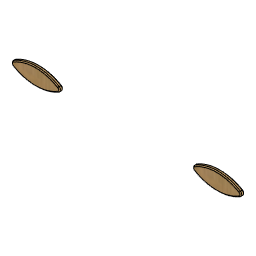
Lamello Bisquit Size 10 Edge SIDE (Autodesk Fusion 360 design; units mm, degrees)
description: Lamello Bisquit
part number: S10
Autodesk Fusion 360 part; units mm, degrees
sketch "Contact Area" plane through (0, 0, 0) normal (0, 0, 1) x (1, 0, 0)
  line L0 (-160, -12.5) -> (160, -12.5)
  line L1 (160, -12.5) -> (160, 12.5)
  line L2 (160, 12.5) -> (-160, 12.5)
  line L3 (-160, 12.5) -> (-160, -12.5)
  line L4 (-160, -12.5) -> (160, 12.5) construction
  line L5 (160, -12.5) -> (-160, 12.5) construction
  dimension "d3" = 320
  dimension "d4" = 25
  constraint horizontal L0
  constraint perpendicular L0 L1
  constraint parallel L0 L2
  constraint parallel L1 L3
  constraint coincident L4 origin
  constraint coincident L5 origin
  measures "d3" distance of L1.end L2.end
  measures "d4" distance of L0.end L1.end
sketch "Egde/SIDE calc" plane through (0, 0, 0) normal (1, 0, 0) x (0, 1, 0)
  line L0 (-50, 18) -> (50, 18)
  line L1 (50, 18) -> (50, 0)
  line L2 (50, 0) -> (-50, 0)
  line L3 (-50, 0) -> (-50, 18)
  line L4 (-50, 18) -> (50, 0) construction
  line L5 (50, 18) -> (-50, 0) construction
  line L6 (12.5, 0) -> (12.5, -40)
  line L7 (12.5, -40) -> (-12.5, -40)
  line L8 (-12.5, -40) -> (-12.5, 0)
  line L9 (-12.5, 0) -> (12.5, 0)
  line L10 (-226.25, 106.25) -> (-213.75, 106.25) construction
  line L11 (-264.0981, 93.7573) -> (-251.5981, 93.7573) construction
  line L12 (-5, 14) -> (5, 14)
  line L13 (5, 14) -> (5, -14)
  line L14 (5, -14) -> (-5, -14)
  line L15 (-5, -14) -> (-5, 14)
  line L16 (-5, 14) -> (5, -14) construction
  line L17 (5, 14) -> (-5, -14) construction
  line L18 (0, -14) -> (0, 14) construction
  line L19 (0, 1.75) -> (0, 22.5) construction
  line L20 (-5, -14) -> (-12.5, -14) construction
  line L21 (0, 0) -> (5, 0) construction
  line L22 (12.5, 0) -> (5, 0) construction
  line L23 (12.5, 0) -> (5, 0) construction
  point P0 (0, 9)
  point P1 (12.5, 0)
  dimension "d20" = 100
  dimension "d21" = 18
  dimension "d23" = 40
  dimension "d24" = 90
  dimension "ReferenceCoord_Calculated" = 12.5
  dimension "OtherSideRefYCoord_Calculated" = 12.5
  dimension "d37" = 12.5
  dimension "d38" = 12.5
  dimension "d39" = 10
  dimension "d40" = 28
  constraint horizontal L0
  constraint perpendicular L0 L1
  constraint parallel L0 L2
  constraint parallel L1 L3
  constraint coincident L4 P0
  constraint coincident L5 P0
  constraint coincident L21.start L2
  constraint coincident L2 L8.end
  constraint coincident L2 P1
  constraint parallel L6 L8
  constraint parallel L2 L7
  constraint coincident L6 P1
  constraint coincident L8 L9.start
  constraint coincident L21.start origin
  constraint horizontal L12
  constraint perpendicular L12 L13
  constraint parallel L12 L14
  constraint parallel L13 L15
  constraint coincident L16 L21.start
  constraint coincident L17 L21.start
  constraint midpoint L14 L18.start
  constraint midpoint L12 L18.end
  constraint coincident L8 L20.end
  constraint perpendicular L8 L20
  constraint midpoint L13 L21.end
  constraint coincident P1 L6.start
  constraint coincident L13 L21.end
  constraint coincident L9 L21.end
  constraint coincident L9 L21.start
  constraint equal L20 L22
  constraint vertical P0 L19.start
  measures "d20" distance of L1.end L2.end
  measures "d21" distance of L0.end L1.end
  measures "d23" distance of L7 L9
  measures "d24" angle of L2 L6
  measures "ReferenceCoord_Calculated" distance of L21.start P1
  measures "OtherSideRefYCoord_Calculated" distance of L21.start L8
  measures "d37" distance of L10.start L10.end
  measures "d38" distance of L11.start L11.end
  measures "d39" distance of L13.end L14.end
  measures "d40" distance of L12.end L13.end
sketch "Pin" plane through (0, 0, 0) normal (0, 0, 1) x (1, 0, 0)
  circle A0 centre (100, 5.75) radius 0.5
  line L0 (160, -12.5) -> (160, 12.5)
  line L1 (160, 12.5) -> (-160, 12.5)
  point P0 (0, -251.5981)
  point P1 (0, -264.0981)
  point P2 (0, -213.75)
  point P3 (0, -226.25)
  dimension "d41" = 1
  dimension "d42" = 60
  dimension "d43" = 12.5
  dimension "OtherSideRefYCoord_CalcProjected" = 12.5
  dimension "ReferenceCoord_CalcProjected" = 12.5
  measures "d41" diameter of A0
  measures "d42" distance of A0.centre L0
  measures "OtherSideRefYCoord_CalcProjected" distance of P0 P1
  measures "ReferenceCoord_CalcProjected" distance of P2 P3
extrude "Extrude1" add sketch "Pin" along normal blind 10 makes body 1
pattern_linear "R-Pattern1" count 2 spacing 200 along (-1, 0, 0) of bodies 1 makes body 2
sketch "Sketch1" plane through (0, 0, 0) normal (0, 0, 1) x (1, 0, 0) in component "Lamello S10 v6"
  line L0 (31.5, -2) -> (-31.5, -2)
  line L1 (-31.5, -2) -> (-31.5, 2)
  line L2 (-31.5, 2) -> (31.5, 2)
  line L3 (31.5, 2) -> (31.5, -2)
  line L4 (31.5, -2) -> (-31.5, 2) construction
  line L5 (-31.5, -2) -> (31.5, 2) construction
  dimension "d8" = 4
  dimension "d9" = 63
  constraint horizontal L0
  constraint perpendicular L0 L1
  constraint parallel L0 L2
  constraint parallel L1 L3
  constraint coincident L4 origin
  constraint coincident L5 origin
  measures "d8" distance of L0 L2
  measures "d9" distance of L1 L3
extrude "Extrude1'" add sketch "Sketch1" along normal mid plane 20 separate body makes body 3 in component "Lamello S10 v6"
sketch "Sketch2" plane through (0, 0, 0) normal (0, 1, 0) x (1, 0, 0) in component "Lamello S10 v6"
  arc A0 (25.0416, 2.5736) -> (-25.0416, 2.5736) centre (0, -39.2308) ccw
  arc A1 (-25.0416, -2.5736) -> (25.0416, -2.5736) centre (0, 39.2308) ccw
  circle A2 centre (-23.5, 0) radius 3
  circle A3 centre (23.5, 0) radius 3
  point P0 (-26.5, 0)
  point P1 (26.5, 0)
  point P2 (0, 9.5)
  point P3 (0, -9.5)
  dimension "d12" = 6
  dimension "d13" = 6
  dimension "d14" = 53
  dimension "d15" = 19
  constraint vertical origin A1.centre
  constraint vertical origin A0.centre
  constraint vertical A0.end A1.start
  constraint vertical A0.start A1.end
  constraint horizontal origin A2.centre
  constraint coincident A0.end A2
  constraint coincident A1.start A2
  constraint tangent A0 A2
  constraint tangent A1 A2
  constraint horizontal origin A3.centre
  constraint coincident A0.start A3
  constraint tangent A0 A3
  constraint coincident A2 P0
  constraint coincident A3 P1
  constraint horizontal origin P0
  constraint horizontal origin P1
  constraint coincident A1 P3
  constraint vertical origin P2
  constraint vertical origin P3
  constraint coincident A0 P2
  measures "d12" diameter of A2
  measures "d13" diameter of A3
  measures "d14" distance of P0 P1
  measures "d15" distance of P2 P3
extrude "Extrude2" add sketch "Sketch2" along normal mid plane 4 separate body makes body 4 in component "Lamello S10 v6"
fillet "Fillet1" radius 1 8 edges at (0, 2, -9.5) (-26.5, 2, 0) (0, 2, 9.5) (26.5, 2, 0) (0, -2, -9.5) (26.5, -2, 0) (0, -2, 9.5) (-26.5, -2, 0) on bodies 4 in component "Lamello S10 v6"
sketch "Sketch4" plane through (0, 0, 0) normal (0, 0, 1) x (1, 0, 0) in component "Lamello S10 v6"
pattern_linear "00000000-0000-0000-0000-000000000000" [suppressed]
component "Lamello S10 v6" placed x (1, 0, 0) y (0, 1, 0) z (0, 0, 1) at (100, 5.75, 0)
component "Lamello S10 v6" placed x (1, 0, 0) y (0, 1, 0) z (0, 0, 1) at (-100, 5.75, 0)
hidden bodies 1 2 3
equation "ContactPatchHeight = 25 mm"
equation "ContactPatchWidth = 320 mm"
equation "d3 = ContactPatchWidth"
equation "d4 = ContactPatchHeight"
equation "X_Coord = if(Count < 1; ContactPatchWidth / 2; DistFromSide1)"
equation "Shift_Y = 0 mm"
equation "Y_Coord = if(ConnectionAngle > 90 deg; OtherSideRefYCoordinate; ReferenceCoord)"
equation "ConnectionAngle = 90 deg" comment "Calculated Automatically!"
equation "AngleForYPositionCalc = if(ConnectionAngle > 90 deg; 180 deg - ConnectionAngle; ConnectionAngle)"
equation "DistFromSide1 = 60 mm"
equation "DistFromSide2 = 60 mm"
equation "PlacingWidth = ContactPatchWidth - DistFromSide1 - DistFromSide2"
equation "MaxDistBetween = 480 mm"
equation "Count = if(MinDistBetween > PlacingWidth; 0; ceil(PlacingWidth / MaxDistBetween))"
equation "MinDistBetween = 96 mm"
equation "OtherSideRefYCoordinate = OtherSideRefYCoord_CalcProjected"
equation "d21 = NestledBoardT"
equation "NestledBoardT = 18 mm" comment "Calculated Automatically!"
equation "d24 = AngleForYPositionCalc"
equation "d37 = ReferenceCoord_Calculated"
equation "d38 = OtherSideRefYCoord_Calculated"
equation "d42 = X_Coord"
equation "d43 = Y_Coord + Shift_Y"
equation "ReferenceCoord = ReferenceCoord_CalcProjected"
equation "Step = PlacingWidth / Count"
equation "d52 = Count + 1"
equation "d54 = -Step"
equation "LamelloLength = 53 mm" comment "Size20 = 56mm; Size10 = 53 mm; Size0 = 47 mm; SizeH9 = 38 mm"
equation "LamelloWidth = 19 mm" comment "Size20 = 23mm; Size10 = 19mm; Size0 = 15 mm; SizeH9 =12 mm"
equation "LamelloThickness = 4 mm" comment "Size20 = 4mm; Size10 = 4 mm; Size0 = 4 mm; SizeH9 = 3mm"
equation "Tolerance = 1 mm" comment "Recommended tolerance for cutting"
equation "GrooveLength = LamelloLength + Tolerance + 9 mm"
equation "GrooveWidth = LamelloWidth + 1 mm"
equation "GrooveThickness = LamelloThickness"
equation "d8 = GrooveThickness"
equation "d9 = GrooveLength"
equation "d10 = GrooveWidth"
equation "d14 = LamelloLength"
equation "d15 = LamelloWidth"
equation "d16 = LamelloThickness"
equation "d72 = Count + 1"
equation "d74 = Step"
named bodies: "Lamello Hole", "Lamello"
